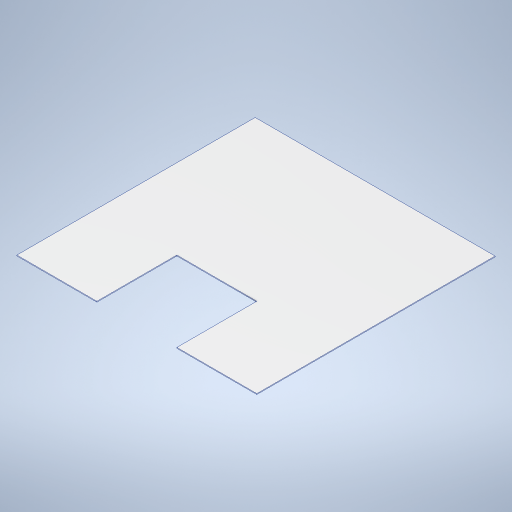
# Autodesk Inventor part: Roof_piece2
Saved by Autodesk Inventor 2023 (Build 270158000, 158)
## iProperties
Created: 2022-12-27
Part Number: Roof_piece2
Material: Aluminum 6061
Document SubType Name: Modeling
Designer: justi
Mass: 790.189 g
Surface Area: 3720.86 cm^2
Volume: 292.663 cm^3
Density: 2.7 g/cm^3
Appearance: Aluminum - Flat
Author: justi
Autodesk Inventor part; units mm, degrees
ref_plane "YZ Plane" through (0, 0, 0) normal (1, 0, 0) x (0, 1, 0)
ref_plane "XZ Plane" through (0, 0, 0) normal (0, 1, 0) x (-1, 0, 0)
ref_plane "XY Plane" through (0, 0, 0) normal (0, 0, 1) x (1, 0, 0)
sketch "Sketch1" plane through (0, 0, 0) normal (0, 1, 0) x (-1, 0, 0)
  line L0 (0, 0) -> (457.2, 0)
  line L1 (457.2, 0) -> (457.2, -454.025)
  line L2 (457.2, -454.025) -> (0, -454.025)
  line L3 (0, -454.025) -> (0, 0)
  line L4 (304.8, 0) -> (152.4, 0)
  line L5 (152.4, 0) -> (152.4, -152.4)
  line L6 (152.4, -152.4) -> (304.8, -152.4)
  line L7 (304.8, -152.4) -> (304.8, 0)
  dimension "d0" = 454.025
  dimension "d1" = 457.2
  dimension "d2" = 152.4
  dimension "d3" = 152.4
  dimension "d4" = 152.4
  constraints: 16 end point, 4 parallel, 2 horizontal, 2 perpendicular, 1 point on line
  measures "d0" distance of L0.end L1.end
  measures "d1" distance of L1.end L2.end
  measures "d2" distance between parallel lines of L1 L7
  measures "d3" distance between parallel lines of L3 L5
  measures "d4" distance of L6.end L4.start
extrude "Extrusion1" add sketch "Sketch1" along normal blind 1.5875 contours L0 L5 L6 L7 L1 L2 L3
body "Solid1"
